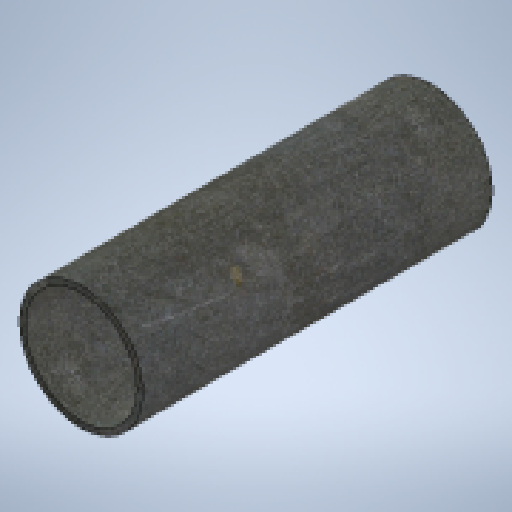
# Autodesk Inventor part: PNS 1733 FDS tube 3_CPY
Saved by Autodesk Inventor 2025.1 (Build 291241020, 241B)
## iProperties
Created: 2025-02-12
Part Number: PNS 1733 FDS tube 3_CPY
Material: Steel
Document SubType Name: Modeling
Designer: user
Mass: 1287.33 g
Surface Area: 1109.67 cm^2
Volume: 163.991 cm^3
Density: 7.85 g/cm^3
Appearance: Plate
Author: pokla
Autodesk Inventor part; units mm, degrees
ref_plane "YZ Plane" through (0, 0, 0) normal (1, 0, 0) x (0, 1, 0)
ref_plane "XZ Plane" through (0, 0, 0) normal (0, 1, 0) x (-1, 0, 0)
ref_plane "XY Plane" through (0, 0, 0) normal (0, 0, 1) x (1, 0, 0)
sketch "Sketch1" plane through (0, 0, 0) normal (0, 1, 0) x (-1, 0, 0)
  circle A0 centre (0, 0) radius 30
  circle A1 centre (0, 0) radius 27
  dimension "d0" = 60
  dimension "d1" = 3
  constraints: 2 centre point, 2 coincident
  measures "d0" diameter of A0
  measures "d1" radial gap between concentric circles of A0 A1
extrude "Extrusion1" add sketch "Sketch1" against normal blind 120
body "Solid1"
